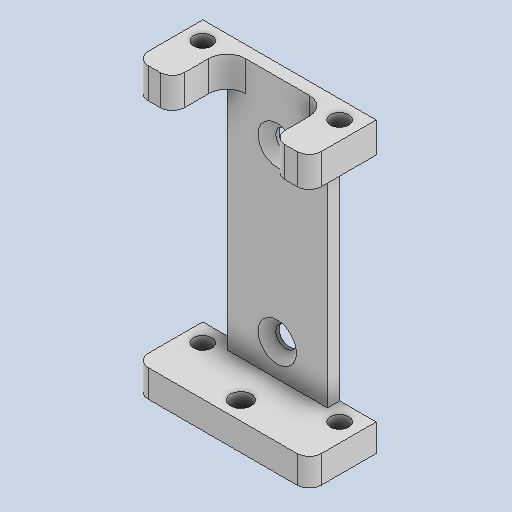
# Autodesk Inventor part: Tension_Bock
Saved by Autodesk Inventor 2024 (Build 280153000, 153)
## iProperties
Created: 2023-07-28
Part Number: Tension_Bock
Material: Generisch
Document SubType Name: Modeling
Designer: aewalder
Density: 1 g/cm^3
Appearance: Vorgabe
Author: aewalder
Autodesk Inventor part; units mm, degrees
ref_plane "YZ Plane" through (0, 0, 0) normal (1, 0, 0) x (0, 1, 0)
ref_plane "XZ Plane" through (0, 0, 0) normal (0, 1, 0) x (-1, 0, 0)
sketch "Sketch1" plane through (0, 0, 0) normal (0, 0, 1) x (1, 0, 0)
  line L0 (-14.25, -23.75) -> (14.25, -23.75)
  line L1 (14.25, -23.75) -> (14.25, 23.75)
  line L2 (14.25, 23.75) -> (-14.25, 23.75)
  line L3 (-14.25, 23.75) -> (-14.25, -23.75)
  line L4 (-14.25, -23.75) -> (14.25, 23.75) construction
  line L5 (14.25, -23.75) -> (-14.25, 23.75) construction
  line L6 (-14.25, 18.75) -> (14.25, 18.75)
  line L7 (-14.25, -19.25) -> (14.25, -19.25)
  line L8 (-8.25, 18.75) -> (-8.25, -19.25)
  line L9 (8.25, 18.75) -> (8.25, -19.25)
  point P0 (0, 0)
  dimension "d0" = 28.5
  dimension "d1" = 47.5
  dimension "d36" = 4.5
  dimension "d37" = 5
  dimension "d38" = 6
  dimension "d39" = 6
  constraints: 20 end point, 8 point on line, 4 perpendicular, 2 midpoint, 2 parallel, 1 horizontal, 1 vertical
  measures "d0" distance between parallel lines of L1 L3
  measures "d1" distance between parallel lines of L0 L2
  measures "d36" distance between parallel lines of L0 L7
  measures "d37" distance between parallel lines of L2 L6
  measures "d38" distance between parallel lines of L3 L8
  measures "d39" distance between parallel lines of L1 L9
extrude "Extrusion1" add sketch "Sketch1" along normal blind 2 contours L3 L7 L1 L0 | L3 L2 L1 L6 | L8 L6 L9 L7
sketch "Sketch2" plane through (0, 0, 2) normal (0, 0, 1) x (1, 0, 0)
  line L0 (-14.25, 23.75) -> (-14.25, -23.75) projected
  line L1 (14.25, -23.75) -> (14.25, 23.75) projected
  line L2 (-14.25, -23.75) -> (14.25, -23.75)
  line L3 (14.25, -23.75) -> (14.25, -19.25)
  line L4 (14.25, -19.25) -> (-14.25, -19.25)
  line L5 (-14.25, -19.25) -> (-14.25, -23.75)
  line L6 (-14.25, 23.75) -> (14.25, 23.75)
  line L7 (14.25, 23.75) -> (14.25, 18.75)
  line L8 (14.25, 18.75) -> (-14.25, 18.75)
  line L9 (-14.25, 18.75) -> (-14.25, 23.75)
  point P0 (0, 0)
  point P1 (14.25, 23.75)
  dimension "d4" = 4.5
  dimension "d19" = 5
  constraints: 16 end point, 4 parallel, 2 horizontal, 2 perpendicular, 2 point on line
  measures "d4" distance between parallel lines of L4 L2
  measures "d19" distance between parallel lines of L6 L8
extrude "Extrusion2" add sketch "Sketch2" along normal blind 9 contours L6 L1 L8 L0 | L4 L1 L2 L0
sketch "Sketch3" plane through (-14.25, -23.75, 0) normal (0, -1, 0) x (1, 0, 0)
  line L0 (0, 11) -> (28.5, 11) construction
  line L1 (14.25, 11) -> (14.25, 0) construction
  line L2 (3, 3) -> (25.5, 3) construction
  line L3 (0, 0) -> (28.5, 0) construction
  point P0 (14.25, 3)
  dimension "d7" = 22.5
  dimension "d8" = 3
  constraints: 4 end point, 2 midpoint, 1 horizontal, 1 point on line, 1 vertical
  measures "d7" distance of L2.end L2.start
  measures "d8" distance between parallel lines of L3 L2
hole "Hole1" at (-11.25, -23.75, 3) at (11.25, -23.75, 3) direction (0, 1, 0) diameter 3 depth 46.5 tip angle 118
sketch "Sketch4" plane through (-14.25, -23.75, 0) normal (0, -1, 0) x (1, 0, 0)
  circle A0 centre (3, 3) radius 1.5 construction
  circle A1 centre (25.5, 3) radius 1.5 construction
  line L0 (3, 3) -> (25.5, 3) construction
  circle A2 centre (14.25, 8) radius 1.7
  line L1 (14.25, 8) -> (14.25, 3) construction
  point P0 (14.25, 0)
  dimension "d40" = 5
  dimension "d41" = 3.4
  constraints: 4 end point, 1 centre point, 1 coincident, 1 horizontal, 1 midpoint, 1 vertical
  measures "d40" distance from line of L0 L1.start
  measures "d41" diameter of A2
extrude "Extrusion3" cut sketch "Sketch4" against normal up to surface (4.5 mm away)
sketch "Sketch6" plane through (-14.25, 23.75, 0) normal (0, 1, 0) x (1, 0, 0)
  line L0 (22.5, -11) -> (6, -11)
  line L1 (6, -11) -> (6, -2)
  line L2 (6, -2) -> (22.5, -2)
  line L3 (22.5, -2) -> (22.5, -11)
  line L4 (22.5, -11) -> (6, -2) construction
  line L5 (6, -11) -> (22.5, -2) construction
  line L6 (14.25, 0) -> (14.25, -11) construction
  line L7 (28.5, -11) -> (0, -11) construction
  line L8 (22.5, -2) -> (6, -2) construction
  circle A0 centre (25.5, -3) radius 1.5 projected
  circle A1 centre (3, -3) radius 1.5 projected
  point P0 (14.25, -6.5)
  point P1 (14.25, -6.5)
  constraints: 14 end point, 4 midpoint, 2 collinear, 2 parallel, 1 horizontal, 1 perpendicular, 1 point on line, 1 vertical
extrude "Extrusion5" cut sketch "Sketch6" against normal up to surface (5 mm away)
fillet "Fillet1" radius 2 6 edges at (-14.25, 21.25, 11) (14.25, 21.25, 11) (-14.25, -21.5, 11) (14.25, -21.5, 11) (-8.25, 21.25, 11) (8.25, 21.25, 11)
fillet "Fillet2" radius 3 2 edges at (-8.25, 21.25, 2) (8.25, 21.25, 2)
ref_plane "Work Plane1" through (-9.075, -7.1151, 3.005) normal (0, 1, 0) x (0, 0, 1)
sketch "Sketch10" plane through (0, 0, 2) normal (0, 0, 1) x (1, 0, 0)
  line L0 (0, 14) -> (0, -14) construction
  point P0 (0, 0)
  point P1 (0, 0)
  dimension "d46" = 28
  constraints: 2 end point, 1 coincident, 1 midpoint, 1 vertical
  measures "d46" distance of L0.start L0.end
hole "Hole2" at (0, 14, 2) at (0, -14, 2) direction (0, 0, -1) diameter 3.4 depth 46.5 tip angle 118 countersink diameter 6.3 countersink angle 90 clearance for "Senkschraube mit Linsenkopf ISO 2010" size "M3" standard "DIN"
equation "\"d1\" = 1.66667 * d0"
equation "\"d39\" = d38"
body "Solid1"
